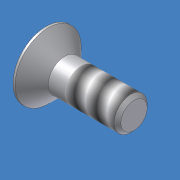
# Autodesk Inventor part: 520 209 112
Saved by Autodesk Inventor 2021.2 (Build 252289000, 289)
## iProperties
_DisabledCommands: 0
Created: 2005-04-22
Part Number: 520 209 112
Material: Allgemein
Vendor: Autodesk Inc.
Document SubType Name: Modeling
Standard: DIN 7991
Designer: SROBAR
Size Designation: M3  x  8
User Status: Veröffentlicht
Engineer: SROBAR
Checked By: AMA
Engr Approved By: AMA
Mfg Approved By: AMA
Density: 1 g/cm^3
Mass: 0.0694516 g
Surface Area: 1.35919 cm^2
Volume: 0.0694516 cm^3
Appearance: Chrom - poliert
EGR: 1
Classification: un/spsc 31161513
Dateiname: 520_209_112
Zeichnungsummer: 520 209 112
Erstellt_am: 07.07.2005
Erstellt_durch: BAR
Geprueft_durch: AMA
Status: Veraltet
Titel: Se-Schr M3 x 8 DIN 7991 A4
Zeichnungsname: 520 209 112
Geprueft_am: 14.07.2005
Zeichnungsnummer: 520 209 112
DOCID: 216990
PDB_IDENT: 520209112
PDB_Name: 520209112
PDB_Ident_Ver: =<PDB_Ident> <PDB_Version>
ROT_Weight: 0.069 g
ROT_Weight_Num: 6.945162233967874e-05
Title: Se-Schr M3 x 8 DIN 7991 A4
Author: SROBAR
Autodesk Inventor part; units mm, degrees
ref_plane "YZ Plane" through (0, 0, 0) normal (1, 0, 0) x (0, 1, 0)
ref_plane "XZ Plane" through (0, 0, 0) normal (0, 1, 0) x (-1, 0, 0)
ref_plane "XY Plane" through (0, 0, 0) normal (0, 0, 1) x (1, 0, 0)
sketch "Skizze1" plane through (0, 0, 0) normal (0, 0, 1) x (1, 0, 0)
  line L0 (8, 0) -> (8, 1.5)
  line L1 (8, 1.5) -> (3.2, 1.5)
  line L2 (3.2, 1.5) -> (2.8933, 1.5)
  line L3 (0, 3) -> (0, 1.1547)
  line L4 (0, 1.1547) -> (1.2, 1.1547)
  line L5 (1.2, 1.1547) -> (1.8667, 0)
  line L6 (1.8667, 0) -> (8, 0)
  line L7 (0, 3) -> (0.2, 3)
  line L8 (0.2, 3) -> (1.7, 1.5)
  line L9 (2.8933, 1.5) -> (1.7, 1.5)
  line L10 (3.2, 1.5) -> (1.7, 1.5) construction
  line L11 (1.7, 1.5) -> (1.7, 1.5)
  line L12 (-12.7, 0) -> (165.1, 0) projected
  line L13 (0, -1.0566) -> (0, 13.7363) projected
  dimension "d0" = 8
  dimension "d1" = 4.8
  dimension "d2" = 1.2
  dimension "d3" = 3
  dimension "d6" = 1.7
  dimension "d7" = 45
  dimension "d8" = 2.3094
  dimension "d9" = 60
  dimension "d10" = 6
  dimension "d11" = 3
  dimension "d12" = 0.3067
  constraints: 24 end point, 4 collinear, 3 parallel
  measures "d0" distance between parallel lines of L3 L0
  measures "d1" distance from line of L1.end L0
  measures "d2" distance from line of L4.end L3
  measures "d3" diameter of L1 L6
  measures "d6" distance from line of L8.end L3
  measures "d7" angle of L8 L6
  measures "d8" diameter of L4 L6
  measures "d9" angle of L5 L6
  measures "d10" diameter of L7 L6
  measures "d11" diameter of L9 L6
  measures "d12" distance of L2.end L1.end
revolve "Körper" add sketch "Skizze1" angle 360 about axis through (1.8667, 0, 0) along (1, 0, 0) contours L6 L5 L4 L3 L7 L8 L9 L2 L1 L0
sketch "Skizze2" plane through (0, 0, 0) normal (-1, 0, 0) x (0, 0, 1)
  circle A0 centre (0, 0) radius 1.1547 projected
  line L0 (0, -3.6) -> (0, 4.8) projected
  line L1 (-3.6, 0) -> (4.8, 0) projected
  line L2 (1.1547, 0) -> (0.5774, -1)
  line L3 (0.5774, -1) -> (-0.5774, -1)
  line L4 (-0.5774, -1) -> (-1.1547, 0)
  line L5 (-1.1547, 0) -> (-0.5774, 1)
  line L6 (-0.5774, 1) -> (0.5774, 1)
  line L7 (0.5774, 1) -> (1.1547, 0)
  point P0 (0, 1.1547)
  constraints: 12 end point, 2 coincident, 2 point on circle, 2 point on line, 12 other
extrude "Loch" add sketch "Skizze2" against normal up to next contours L7 A0 | A0 L2 | L6 L0 A0 | A0 L0 L3 | L0 L6 A0 | A0 L3 L0 | L4 A0 | A0 L5
thread "Gewinde" size "M3x0.5" designation "M3" class "6g" standard "ANSI Metrisches M Profil" length 4.8
chamfer "Fase1" distance 0.3067 distance2 0.3067 1 edges at (8, -1.5, 0) measured on face at (8, -0.8298, -0.2045)
equation "\"d0\" = NLG"
equation "\"d1\" = GEL"
equation "\"d2\" = INTI"
equation "\"d3\" = GD"
equation "\"d6\" = KOH"
equation "\"d7\" = 0.5 * SEWI"
equation "\"d8\" = 1.1547 * SW"
equation "\"d10\" = KOD"
equation "\"d11\" = BDM"
equation "\"d12\" = GAL"
equation "\"d15\" = GEL"
equation "\"d17\" = -0.5 * SPD + 0.5 * GD"
equation "\"d18\" = GUL"
equation "\"NLG\" = 8"
equation "\"INTI\" = 1.2"
equation "\"GEL\" = 4.8"
equation "\"GAL\" = 0.61345 * TPU"
equation "\"KOH\" = 1.7"
equation "\"KOD\" = 6"
equation "\"GUL\" = 0.61345 * TPU"
equation "\"SPD\" = NND - 1.2269 * TPU"
equation "\"BDM\" = NND"
equation "\"GD\" = NND"
equation "\"SEWI\" = 90deg"
equation "\"SW\" = 2"
equation "\"NND\" = 3"
equation "\"EPV\" = 3.2"
equation "\"E0\" = 1.155 * SW"
equation "\"THREADDIA\" = 3"
equation "\"TPU\" = 0.5"
equation "\"GD1\" = THREADDIA - 1.2269 * TPU"
equation "\"PTC\" = TPU"
equation "\"TOA\" = 30deg"
